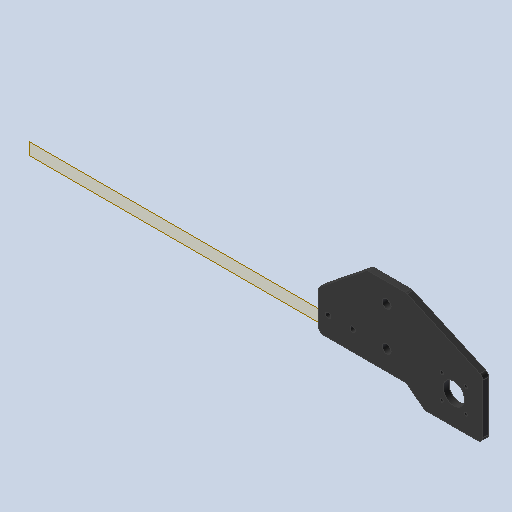
# Autodesk Inventor part: 6MM_ENDPLATE_FLOATINGSIDE
Saved by Autodesk Inventor 2025.2 (Build 292293000, 293)
## iProperties
Created: 2026-02-06
Part Number: 6MM_ENDPLATE_FLOATINGSIDE
Material: Generic
Document SubType Name: Modeling
Designer: composite
Density: 1 g/cm^3
Appearance: Default
Author: composite
Autodesk Inventor part; units mm, degrees
ref_plane "YZ Plane" through (0, 0, 0) normal (1, 0, 0) x (0, 1, 0)
ref_plane "XZ Plane" through (0, 0, 0) normal (0, 1, 0) x (-1, 0, 0)
ref_plane "XY Plane" through (0, 0, 0) normal (0, 0, 1) x (1, 0, 0)
ref_plane "Work Plane1" through (0, -22.3046, 0) normal (0, 0, 1) x (1, 0, 0)
sketch "Sketch1" plane through (0, -22.3046, 0) normal (0, 0, 1) x (1, 0, 0)
  circle A0 centre (356.5, 45.63) radius 4.5 projected
  circle A1 centre (401.93, -22.94) radius 2.5 projected
  circle A2 centre (410.6508, 15.4792) radius 2.25 projected
  circle A3 centre (410.6508, -14.2192) radius 2.25 projected
  circle A4 centre (440.3492, -14.2192) radius 2.25 projected
  circle A5 centre (449.07, 24.2) radius 2.5 projected
  circle A6 centre (440.3492, 15.4792) radius 2.25 projected
  circle A7 centre (425.5, 0.63) radius 11 projected
  circle A8 centre (296.5, 5.63) radius 2.75 projected
  circle A9 centre (321.5, 5.63) radius 2.75 projected
  circle A10 centre (449.07, -22.94) radius 2.5 projected
  circle A11 centre (401.93, 24.2) radius 2.5 projected
  circle A12 centre (356.5, 5.63) radius 4.5 projected
  arc A13 (455.2, 27.0928) -> (452.2463, 31.6549) centre (450.2, 27.0928) ccw projected
  line L0 (377.4763, 65.1921) -> (452.2463, 31.6549) projected
  arc A14 (377.4763, 65.1921) -> (375.43, 65.63) centre (375.43, 60.63) ccw projected
  line L1 (338.2539, 65.63) -> (375.43, 65.63) projected
  arc A15 (338.2539, 65.63) -> (335.1304, 64.5343) centre (338.2539, 60.63) ccw projected
  line L2 (288.3765, 27.1312) -> (335.1304, 64.5343) projected
  arc A16 (288.3765, 27.1312) -> (286.5, 23.2269) centre (291.5, 23.2269) ccw projected
  line L3 (286.5, -9.37) -> (286.5, 23.2269) projected
  arc A17 (286.5, -9.37) -> (291.5, -14.37) centre (291.5, -9.37) ccw projected
  line L4 (374.8127, -14.37) -> (291.5, -14.37) projected
  arc A18 (377.8423, -15.3924) -> (374.8127, -14.37) centre (374.8127, -19.37) ccw projected
  line L5 (394.4577, -28.0476) -> (377.8423, -15.3924) projected
  arc A19 (394.4577, -28.0476) -> (397.4873, -29.07) centre (397.4873, -24.07) ccw projected
  line L6 (450.2, -29.07) -> (397.4873, -29.07) projected
  arc A20 (450.2, -29.07) -> (455.2, -24.07) centre (450.2, -24.07) ccw projected
  line L7 (455.2, 27.0928) -> (455.2, -24.07) projected
  circle A21 centre (425.5, 0.63) radius 17.5 construction
  circle A22 centre (413.1256, 13.0044) radius 1.7
  circle A23 centre (425.5, 0.63) radius 17.5 construction
  circle A24 centre (413.1256, -11.7444) radius 1.7
  circle A25 centre (425.5, 0.63) radius 17.5 construction
  circle A26 centre (437.8744, -11.7444) radius 1.7
  circle A27 centre (425.5, 0.63) radius 17.5 construction
  circle A28 centre (437.8744, 13.0044) radius 1.7
  point P0 (0, 22.3046)
  dimension "d0" = 35
  dimension "d1" = 3.4
  dimension "d4" = 360
  constraints: 4 centre point, 1 coincident, 1 vertical alignment, 29 other
  measures "d1" diameter of A22
extrude "Extrusion1" add sketch "Sketch1" along normal blind 6 contours A1 | A2 A22 | A3 A24 | A4 A26 | A5 | A6 A28 | A10 | A11 | L7 A20 L6 A19 L5 A18 L4 A17 L3 A16 L2 A15 L1 A14 L0 A13 picked at (410.1303, 16.2077) picked at (410.1303, -14.9477) picked at (440.8941, -14.9263) picked at (440.8941, 16.1863)
body "Solid1"
